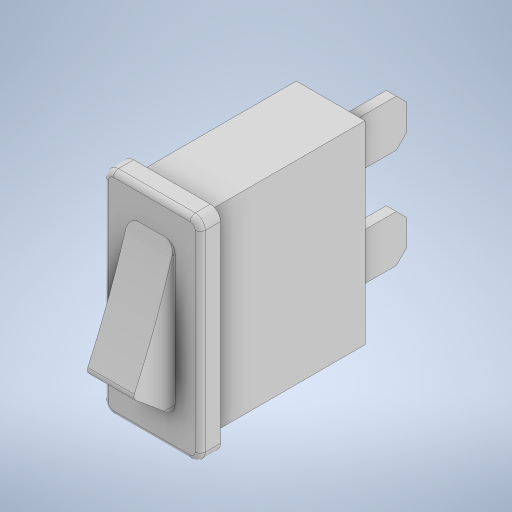
# Autodesk Inventor part: RockerSwitch
Saved by Autodesk Inventor 2023 (Build 270158000, 158)
## iProperties
Created: 2023-11-27
Part Number: RockerSwitch
Material: Generic
Document SubType Name: Modeling
Designer: LattePanda
Density: 1 g/cm^3
Appearance: Default
Author: LattePanda
Autodesk Inventor part; units mm, degrees
ref_plane "YZ Plane" through (0, 0, 0) normal (1, 0, 0) x (0, 1, 0)
ref_plane "XZ Plane" through (0, 0, 0) normal (0, 1, 0) x (-1, 0, 0)
sketch "Base" plane through (0, 0, 0) normal (0, 0, 1) x (1, 0, 0)
  line L0 (-3.4, 9.6) -> (3.4, 9.6)
  line L1 (3.4, 9.6) -> (3.4, -9.6)
  line L2 (3.4, -9.6) -> (-3.4, -9.6)
  line L3 (-3.4, -9.6) -> (-3.4, 9.6)
  line L4 (-4.76, 0) -> (4.76, 0) construction
  line L5 (0, -13.44) -> (0, 13.44) construction
  point P0 (0, 0)
  point P1 (0, 9.6)
  point P2 (-3.4, 0)
  dimension "d0" = 6.8
  dimension "d1" = 19.2
  constraints: 8 end point, 2 midpoint, 2 parallel, 2 point on line, 1 horizontal, 1 perpendicular
  measures "d0" distance of L0.start L0.end
  measures "d1" distance of L2.end L0.start
extrude "BaseFeature" add sketch "Base" along normal blind 17.7
sketch "Mount" plane through (0, 0, 17.7) normal (0, 0, 1) x (1, 0, 0)
  line L0 (-4.8, 10.5) -> (4.8, 10.5)
  line L1 (4.8, 10.5) -> (4.8, -10.5)
  line L2 (4.8, -10.5) -> (-4.8, -10.5)
  line L3 (-4.8, -10.5) -> (-4.8, 10.5)
  line L4 (3.4, -9.6) -> (3.4, 9.6) construction
  line L5 (3.4, 0) -> (4.8, 0) construction
  line L6 (-3.4, -9.6) -> (3.4, -9.6) construction
  line L7 (0, -9.6) -> (0, -10.5) construction
  dimension "d13" = 9.6
  dimension "d14" = 21
  constraints: 12 end point, 5 perpendicular, 4 midpoint, 1 horizontal
  measures "d13" distance of L1.end L2.end
  measures "d14" distance of L0.end L1.end
extrude "MountFeature" add sketch "Mount" against normal blind 2
sketch "Sketch3" plane through (0, 0, 17.7) normal (0, 0, 1) x (1, 0, 0)
  line L0 (-2.3, -7.45) -> (2.3, -7.45)
  line L1 (-2.3, 7.45) -> (-2.3, -7.45)
  line L2 (2.3, 7.45) -> (-2.3, 7.45)
  line L3 (2.3, -7.45) -> (2.3, 7.45)
  line L4 (-4.8, 10.5) -> (-4.8, -10.5) projected
  line L5 (0, 0) -> (0, 10.5) construction
  line L6 (-4.8, 10.5) -> (4.8, 10.5) projected
  line L7 (-6.72, 0) -> (6.72, 0) construction
  point P0 (0, 7.45)
  point P1 (-2.3, 0)
  dimension "d22" = 14.9
  dimension "d23" = 4.6
  constraints: 10 end point, 3 midpoint, 3 perpendicular, 2 point on line, 1 parallel
  measures "d22" distance of L1.start L0.start
  measures "d23" distance of L2.start L1.start
extrude "Extrusion3" add sketch "Sketch3" along normal blind 4.2
fillet "Fillet4" radius 1 4 edges at (-2.3, 7.45, 19.8) (2.3, 7.45, 19.8) (-2.3, -7.45, 19.8) (2.3, -7.45, 19.8)
sketch "Sketch4" plane through (2.3, -7.45, 17.7) normal (1, 0, 0) x (0, 0, -1)
  line L0 (0, 0) -> (-4.2, 0) projected
  line L1 (-4.2, 14.9) -> (-4.2, 0) projected
  arc A0 (0, 0) -> (-4.2, 3.5647) centre (-50.9891, -55.8203) ccw
  line L2 (0, 0) -> (0, 14.9) projected
  arc A1 (-4.2, 3.5647) -> (0, 14.9) centre (-72.7661, 35.4157) ccw
  line L3 (0, 14.9) -> (-4.2, 14.9) projected
  point P0 (17.7, 7.45)
  constraints: 4 point on circle, 2 centre point, 1 point on line
extrude "Extrusion4" cut sketch "Sketch4" against normal through all contours L0 L1 A0 | L1 L3 A1
fillet "Fillet1" radius 0.5 1 edges at (0, -3.8853, 21.9)
fillet "Fillet2" radius 1 4 edges at (4.8, -10.5, 16.7) (4.8, 10.5, 16.7) (-4.8, 10.5, 16.7) (-4.8, -10.5, 16.7)
fillet "Fillet3" radius 0.5 4 edges at (0, -10.5, 17.7) (4.8, 0, 17.7) (0, 10.5, 17.7) (-4.8, 0, 17.7)
sketch "Sketch6" plane through (-3.4, -9.6, 0) normal (-1, 0, 0) x (0, 0, 1)
  line L0 (0, 0) -> (0, 19.2) construction
  line L1 (0, 9.6) -> (0, 19.2)
  line L2 (0, 9.6) -> (15.7, 9.6) construction
  line L3 (15.7, 0) -> (15.7, 19.2) projected
  line L4 (0, 16.8553) -> (-7, 16.8553)
  line L5 (-7, 16.8553) -> (-7, 12.233)
  line L6 (-7, 12.233) -> (0, 12.233)
  line L7 (0, 12.233) -> (0, 16.8553)
  line L8 (0, 14.5441) -> (-7, 14.5441) construction
  line L9 (0, 2.3447) -> (-7, 2.3447)
  line L10 (-7, 2.3447) -> (-7, 6.967)
  line L11 (-7, 6.967) -> (0, 6.967)
  line L12 (0, 6.967) -> (0, 2.3447)
  dimension "d16" = 7
  constraints: 22 end point, 4 symmetric about line, 3 midpoint, 2 parallel, 1 horizontal, 1 perpendicular, 1 point on line, 1 vertical
  measures "d16" distance of L4.start L4.end
ref_plane "Work Plane1" through (0, -9.6, 0) normal (-1, 0, 0) x (0, 0, 1)
sketch "Sketch7" plane through (0, -9.6, 0) normal (-1, 0, 0) x (0, 0, 1)
  line L0 (0, 16.8553) -> (-7, 16.8553) projected
  line L1 (-7, 16.8553) -> (-7, 12.233) projected
  line L2 (-7, 12.233) -> (0, 12.233) projected
  line L3 (0, 19.2) -> (0, 0) projected
  line L4 (-7, 6.967) -> (0, 6.967) projected
  line L5 (-7, 2.3447) -> (-7, 6.967) projected
  line L6 (0, 2.3447) -> (-7, 2.3447) projected
  point P0 (0, 9.6)
extrude "Extrusion5" add sketch "Sketch7" along normal mid plane 1
chamfer "Chamfer1" distance 1 angle 45 4 edges at (0, 7.2553, -7) (0, 2.633, -7) (0, -2.633, -7) (0, -7.2553, -7)
body "Solid1"
